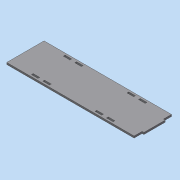
# Autodesk Inventor part: slider-holder_side
Saved by Autodesk Inventor 2016 SP1 (Build 200210100, 210)
## iProperties
Created: 2016-03-30
Part Number: slider-holder_side
Material: Generic
Document SubType Name: Modeling
Designer: Mohamed A.
Density: 1 g/cm^3
Appearance: Default
Author: Mohamed A.
Autodesk Inventor part; units mm, degrees
ref_plane "YZ Plane" through (0, 0, 0) normal (1, 0, 0) x (0, 1, 0)
ref_plane "XZ Plane" through (0, 0, 0) normal (0, 1, 0) x (-1, 0, 0)
ref_plane "XY Plane" through (0, 0, 0) normal (0, 0, 1) x (1, 0, 0)
sketch "Sketch1" plane through (0, 0, 0) normal (0, 0, 1) x (1, 0, 0)
  line L0 (0, 6) -> (211.4, 6)
  line L1 (211.4, 6) -> (211.4, -53)
  line L2 (211.4, -53) -> (0, -53)
  line L3 (0, -53) -> (0, 6)
  line L4 (214.4, 3) -> (214.4, 0) projected
  line L5 (37.85, -53) -> (0, -53) projected
  line L6 (0, 6) -> (211.4, 6) projected
  line L7 (211.4, 3) -> (211.4, 6) projected
  line L8 (0, -53) -> (0, -56)
  line L9 (0, -56) -> (211.4, -56)
  line L10 (211.4, -56) -> (211.4, -53)
  line L11 (211.4, -42.7143) -> (214.4, -42.7143)
  line L12 (214.4, -42.7143) -> (214.4, -7.2857)
  line L13 (214.4, -7.2857) -> (211.4, -7.2857)
  line L14 (-8.1633, -25) -> (265.4045, -25) construction
  line L15 (37.85, 3) -> (48.85, 3) projected
  line L16 (37.85, 3) -> (37.85, 0) projected
  line L17 (48.85, 0) -> (37.85, 0) projected
  line L18 (48.85, 3) -> (48.85, 0) projected
  line L19 (56.85, 3) -> (67.85, 3) projected
  line L20 (56.85, 3) -> (56.85, 0) projected
  line L21 (67.85, 0) -> (56.85, 0) projected
  line L22 (67.85, 3) -> (67.85, 0) projected
  line L23 (143.55, 3) -> (154.55, 3) projected
  line L24 (143.55, 3) -> (143.55, 0) projected
  line L25 (154.55, 0) -> (143.55, 0) projected
  line L26 (154.55, 3) -> (154.55, 0) projected
  line L27 (162.55, 3) -> (173.55, 3) projected
  line L28 (162.55, 3) -> (162.55, 0) projected
  line L29 (173.55, 0) -> (162.55, 0) projected
  line L30 (173.55, 3) -> (173.55, 0) projected
  line L31 (162.55, -50) -> (173.55, -50) projected
  line L32 (162.55, -50) -> (162.55, -53) projected
  line L33 (173.55, -53) -> (162.55, -53) projected
  line L34 (173.55, -50) -> (173.55, -53) projected
  line L35 (143.55, -50) -> (154.55, -50) projected
  line L36 (143.55, -50) -> (143.55, -53) projected
  line L37 (154.55, -53) -> (143.55, -53) projected
  line L38 (154.55, -50) -> (154.55, -53) projected
  line L39 (56.85, -50) -> (67.85, -50) projected
  line L40 (56.85, -50) -> (56.85, -53) projected
  line L41 (67.85, -53) -> (56.85, -53) projected
  line L42 (67.85, -50) -> (67.85, -53) projected
  line L43 (37.85, -50) -> (48.85, -50) projected
  line L44 (37.85, -50) -> (37.85, -53) projected
  line L45 (48.85, -53) -> (37.85, -53) projected
  line L46 (48.85, -50) -> (48.85, -53) projected
  line L47 (143.55, -53) -> (154.55, -53)
  line L48 (154.55, -53) -> (154.55, -50)
  line L49 (154.55, -50) -> (143.55, -50)
  line L50 (143.55, -50) -> (143.55, -53)
  line L51 (162.55, -53) -> (173.55, -53)
  line L52 (173.55, -53) -> (173.55, -50)
  line L53 (173.55, -50) -> (162.55, -50)
  line L54 (162.55, -50) -> (162.55, -53)
  line L55 (56.85, -53) -> (67.85, -53)
  line L56 (67.85, -53) -> (67.85, -50)
  line L57 (67.85, -50) -> (56.85, -50)
  line L58 (56.85, -50) -> (56.85, -53)
  line L59 (48.85, -53) -> (37.85, -53)
  line L60 (37.85, -53) -> (37.85, -50)
  line L61 (37.85, -50) -> (48.85, -50)
  line L62 (48.85, -50) -> (48.85, -53)
  line L63 (211.4, -56) -> (0, -56)
  line L64 (0, -56) -> (0, -53)
  line L65 (0, -53) -> (211.4, -53)
  line L66 (211.4, -53) -> (211.4, -56)
  line L67 (154.55, 0) -> (162.55, 3) construction
  line L68 (154.55, 3) -> (162.55, 0) construction
  line L69 (48.85, 3) -> (56.85, 0) construction
  line L70 (48.85, 0) -> (56.85, 3) construction
  line L71 (48.85, -50) -> (56.85, -53) construction
  line L72 (48.85, -53) -> (56.85, -50) construction
  line L73 (154.55, -53) -> (162.55, -50) construction
  line L74 (154.55, -50) -> (162.55, -53) construction
  circle A0 centre (158.55, 1.5) radius 1.4
  circle A1 centre (52.85, 1.5) radius 1.4
  circle A2 centre (52.85, -51.5) radius 1.4
  circle A3 centre (158.55, -51.5) radius 1.4
  point P0 (0, 0)
  dimension "d0" = 3
  dimension "d1" = 3
  dimension "d2" = 62
  dimension "d3" = 31
  dimension "d4" = 35.4286
  dimension "d7" = 2.8
  dimension "d8" = 2.8
  dimension "d9" = 2.8
  dimension "d10" = 2.8
  constraints: 78 end point, 19 parallel, 8 horizontal, 8 perpendicular, 4 centre point, 4 midpoint, 4 point on line, 3 collinear, 2 vertical, 1 other
  measures "d0" distance of L5.end L8.end
  measures "d1" distance between parallel lines of L12 L1
  measures "d2" distance between parallel lines of L9 L6
  measures "d3" distance between parallel lines of L14 L6
  measures "d4" distance between parallel lines of L11 L13
  measures "d7" diameter of A0
  measures "d8" diameter of A1
  measures "d9" diameter of A2
  measures "d10" diameter of A3
extrude "Extrusion1" add sketch "Sketch1" along normal blind 3 contours L0 L1 L2 L34 L31 L32 L38 L35 L36 L42 L39 L40 L46 L43 L44 L3 | L2 L10 L9 L8 | L13 L12 L11 L1
equation "\"d3\" = 0.5 * d2"
equation "\"d4\" = 0.571429 * d2"
body "Solid1"
